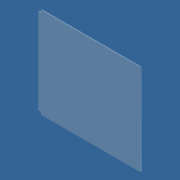
# Autodesk Inventor part: base plate
Saved by Autodesk Inventor 2012 (Build 160160000, 160)
## iProperties
Created: 2012-03-15
Part Number: base plate
Material: Polycarbonate, Clear
Document SubType Name: Modeling
Designer: Ed
Mass: 1928.1 g
Surface Area: 5188.7 cm^2
Volume: 1606.75 cm^3
Density: 1.2 g/cm^3
Author: Ed
Autodesk Inventor part; units mm, degrees
ref_plane "YZ Plane" through (0, 0, 0) normal (1, 0, 0) x (0, 1, 0)
ref_plane "XZ Plane" through (0, 0, 0) normal (0, 1, 0) x (-1, 0, 0)
ref_plane "XY Plane" through (0, 0, 0) normal (0, 0, 1) x (1, 0, 0)
sketch "Sketch1" plane through (0, 0, 0) normal (0, 0, 1) x (1, 0, 0)
  line L0 (0, 0) -> (533.4, 0)
  line L1 (533.4, 0) -> (533.4, 474.98)
  line L2 (533.4, 474.98) -> (0, 474.98)
  line L3 (0, 474.98) -> (0, 0)
  line L4 (0, 0) -> (12.7, 0)
  line L5 (12.7, 0) -> (12.7, 12.7)
  line L6 (12.7, 12.7) -> (0, 12.7)
  line L7 (0, 12.7) -> (0, 0)
  line L8 (0, 474.98) -> (12.7, 474.98)
  line L9 (12.7, 474.98) -> (12.7, 462.28)
  line L10 (12.7, 462.28) -> (0, 462.28)
  line L11 (0, 462.28) -> (0, 474.98)
  dimension "d0" = 474.98
  dimension "d1" = 533.4
  dimension "d2" = 12.7
  constraints: 24 end point, 6 parallel, 3 equal length, 3 horizontal, 3 perpendicular
  measures "d0" distance of L2.end L0.start
  measures "d1" distance of L0.start L0.end
  measures "d2" distance of L8.end L9.end
extrude "Extrusion1" add sketch "Sketch1" along normal blind 6.35 contours L5 L6 L3 L10 L9 L2 L1 L0
body "Solid1"
